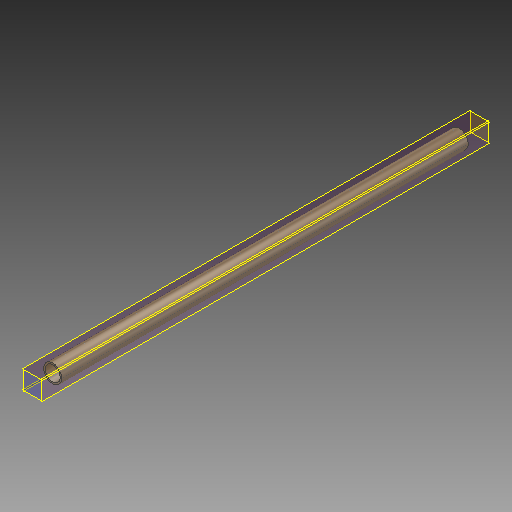
# Autodesk Inventor part: Pipe6
Saved by Autodesk Inventor 2018 (Build 220112000, 112)
## iProperties
Created: 2017-09-13
Part Number: Pipe6
Material: 鋼、炭素鋼
Document SubType Name: Modeling
Designer: mura5
Density: 7.85 g/cm^3
Appearance: 半つや出し
Mass: 860.224 g
Surface Area: 956.491 cm^2
Volume: 109.583 cm^3
Author: mura5
Autodesk Inventor part; units mm, degrees
ref_plane "XY Plane" through (0, 0, 0) normal (0, 0, 1) x (1, 0, 0)
sketch "スケッチ1" plane through (0, 0, 0) normal (0, 0, 1) x (1, 0, 0)
  circle A0 centre (0, 0) radius 13.6
  circle A1 centre (0, 0) radius 11.3
  dimension "d0" = 27.2
  dimension "d1" = 2.3
  constraints: 2 centre point, 1 coincident
  measures "d0" diameter of A0
  measures "d1" radial gap between concentric circles of A0 A1
extrude "押し出し1" add sketch "スケッチ1" along normal mid plane 609.0667
ref_plane "作業平面1" through (13.6, 0, 0) normal (1, 0, 0) x (0, 1, 0)
ref_plane "作業平面2" through (-13.6, 0, 0) normal (-1, 0, 0) x (0, -1, 0)
ref_plane "作業平面3" through (0, 13.6, 0) normal (0, 1, 0) x (-1, 0, 0)
ref_plane "作業平面4" through (0, -13.6, 0) normal (0, -1, 0) x (1, 0, 0)
